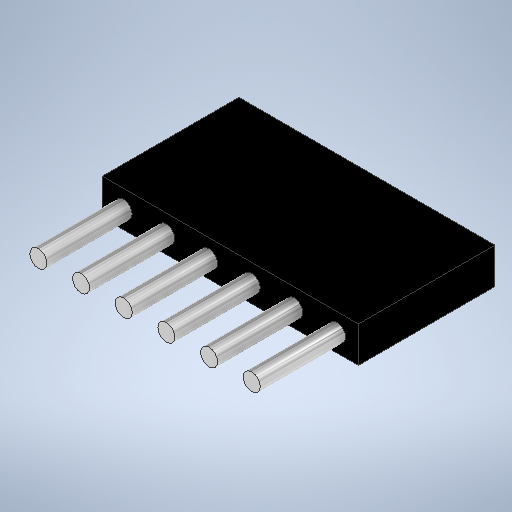
# Autodesk Inventor part: connector
Saved by Autodesk Inventor 2025.2 (Build 292293000, 293)
## iProperties
Created: 2025-04-04
Part Number: connector
Material: Generic
Document SubType Name: Modeling
Designer: joaki
Density: 1 g/cm^3
Appearance: Default
Author: joaki
Autodesk Inventor part; units mm, degrees
ref_plane "YZ Plane" through (0, 0, 0) normal (1, 0, 0) x (0, 1, 0)
ref_plane "XZ Plane" through (0, 0, 0) normal (0, 1, 0) x (-1, 0, 0)
ref_plane "XY Plane" through (0, 0, 0) normal (0, 0, 1) x (1, 0, 0)
sketch "Sketch1" plane through (0, 0, 0) normal (0, 1, 0) x (-1, 0, 0)
  line L0 (8.9303, 10.1039) -> (-6.0697, 10.1039)
  line L1 (-6.0697, 10.1039) -> (-6.0697, 2.1039)
  line L2 (-6.0697, 2.1039) -> (8.9303, 2.1039)
  line L3 (8.9303, 2.1039) -> (8.9303, 10.1039)
  point P0 (0, 0)
  point P1 (1.4303, 10.1039)
  dimension "d0" = 15
  dimension "d1" = 8
  constraints: 8 end point, 2 parallel, 1 horizontal, 1 midpoint, 1 perpendicular
  measures "d0" distance between parallel lines of L1 L3
  measures "d1" distance from line of point (1.43, 10.104) L2
extrude "Extrusion1" add sketch "Sketch1" along normal blind 2.1
sketch "Sketch2" plane through (-8.9303, 0, 10.1039) normal (0, 0, 1) x (1, 0, 0)
  circle A0 centre (1.25, 1.05) radius 0.5
  circle A1 centre (3.75, 1.05) radius 0.5
  circle A2 centre (6.25, 1.05) radius 0.5
  circle A3 centre (8.75, 1.05) radius 0.5
  circle A4 centre (11.25, 1.05) radius 0.5
  circle A5 centre (13.75, 1.05) radius 0.5
  line L0 (0, 2.1) -> (15, 2.1) projected
  line L1 (15, 0) -> (0, 0) projected
  line L2 (7.5, 0) -> (7.5, 2.1)
  point P0 (8.9303, 0)
  dimension "d4" = 1
  dimension "d5" = 1
  dimension "d6" = 1
  dimension "d7" = 1
  dimension "d8" = 1
  dimension "d9" = 1
  dimension "d10" = 1.05
  dimension "d11" = 1.05
  dimension "d12" = 1.05
  dimension "d13" = 1.05
  dimension "d14" = 1.05
  dimension "d15" = 1.05
  dimension "d16" = 1.25
  dimension "d17" = 2.5
  dimension "d18" = 2.5
  dimension "d19" = 1.25
  dimension "d20" = 2.5
  dimension "d21" = 2.5
  constraints: 6 centre point, 2 end point, 2 midpoint
  measures "d4" diameter of A0
  measures "d5" diameter of A1
  measures "d6" diameter of A2
  measures "d7" diameter of A3
  measures "d8" diameter of A4
  measures "d9" diameter of A5
  measures "d10" distance from line of L0 A0.centre
  measures "d11" distance from line of L0 A1.centre
  measures "d12" distance from line of L0 A2.centre
  measures "d13" distance from line of L0 A3.centre
  measures "d14" distance from line of L0 A4.centre
  measures "d15" distance from line of L0 A5.centre
  measures "d16" distance from line of A2.centre L2
  measures "d17" distance of A1.centre A2.centre
  measures "d18" distance of A0.centre A1.centre
  measures "d19" distance from line of L2 A3.centre
  measures "d20" distance of A3.centre A4.centre
  measures "d21" distance of A4.centre A5.centre
extrude "Extrusion2" add sketch "Sketch2" along normal blind 5
body "Solid1"
